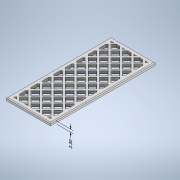
# Autodesk Inventor part: Part_B3
Saved by Autodesk Inventor 2022.6 (Build 266554010, 554A)
## iProperties
Created: 2025-05-15
Part Number: Part_B3
Material: Generic
Document SubType Name: Modeling
Designer: khinm
Density: 1 g/cm^3
Appearance: Default
Author: khinm
Autodesk Inventor part; units mm, degrees
ref_plane "YZ Plane" through (0, 0, 0) normal (1, 0, 0) x (0, 1, 0)
ref_plane "XZ Plane" through (0, 0, 0) normal (0, 1, 0) x (-1, 0, 0)
ref_plane "XY Plane" through (0, 0, 0) normal (0, 0, 1) x (1, 0, 0)
sketch "Sketch1" plane through (0, 0, 0) normal (0, 1, 0) x (-1, 0, 0)
  line L0 (27.4, -64.9) -> (-27.4, -64.9)
  line L1 (-27.4, -64.9) -> (-27.4, 64.9)
  line L2 (-27.4, 64.9) -> (27.4, 64.9)
  line L3 (27.4, 64.9) -> (27.4, -64.9)
  point P0 (0, 0)
  point P1 (27.4, 0)
  point P2 (0, -64.9)
  dimension "d0" = 54.8
  dimension "d1" = 129.8
  constraints: 8 end point, 2 midpoint, 2 parallel, 1 horizontal, 1 horizontal alignment, 1 perpendicular, 1 vertical alignment
  measures "d0" distance of L1.end L2.end
  measures "d1" distance between parallel lines of L2 L0
extrude "Extrusion1" add sketch "Sketch1" along normal mid plane 3.3
sketch "Sketch2" plane through (0, 1.65, 0) normal (0, 1, 0) x (1, 0, 0)
  line L0 (-27.4, -64.9) -> (27.4, -64.9) projected
  line L1 (-27.4, 64.9) -> (-27.4, -64.9) projected
  line L2 (22.4, 59.9) -> (22.4, -59.9)
  line L3 (22.4, -59.9) -> (-22.4, -59.9)
  line L4 (27.4, 64.9) -> (-27.4, 64.9) projected
  line L5 (27.4, -64.9) -> (27.4, 64.9) projected
  line L6 (22.4, 59.9) -> (-22.4, 59.9)
  line L7 (-22.4, -59.9) -> (22.4, -59.9)
  line L8 (22.4, -59.9) -> (22.4, 59.9)
  line L9 (21.2132, -30.0452) -> (22.4, -31.232)
  line L10 (16.2635, -34.9949) -> (21.2132, -39.9447)
  line L11 (-4.9497, -56.2081) -> (-1.2579, -59.9)
  line L12 (-7.0711, -58.3294) -> (-5.5005, -59.9)
  line L13 (14.1421, -37.1162) -> (19.0919, -42.066)
  line L14 (21.2132, -44.1873) -> (22.4, -45.3741)
  line L15 (9.1924, -42.066) -> (14.1421, -47.0157)
  line L16 (16.2635, -49.137) -> (21.2132, -54.0868)
  line L17 (7.0711, -44.1873) -> (12.0208, -49.137)
  line L18 (2.1213, -49.137) -> (7.0711, -54.0868)
  line L19 (9.1924, -56.2081) -> (12.8843, -59.9)
  line L20 (0, -51.2584) -> (4.9497, -56.2081)
  line L21 (7.0711, -58.3294) -> (8.6416, -59.9)
  line L22 (21.2132, -15.903) -> (22.4, -17.0898)
  line L23 (16.2635, -20.8528) -> (21.2132, -25.8025)
  line L24 (14.1421, -22.9741) -> (19.0919, -27.9238)
  line L25 (9.1924, -27.9238) -> (14.1421, -32.8736)
  line L26 (7.0711, -30.0452) -> (12.0208, -34.9949)
  line L27 (2.1213, -34.9949) -> (7.0711, -39.9447)
  line L28 (0, -37.1162) -> (4.9497, -42.066)
  line L29 (-4.9497, -42.066) -> (0, -47.0157)
  line L30 (-7.0711, -44.1873) -> (-2.1213, -49.137)
  line L31 (-12.0208, -49.137) -> (-7.0711, -54.0868)
  line L32 (-21.2132, -44.1873) -> (-16.2635, -49.137)
  line L33 (-14.1421, -51.2584) -> (-9.1924, -56.2081)
  line L34 (-22.4, -52.9) -> (-21.2132, -54.0868)
  line L35 (-19.0919, -56.2081) -> (-15.4, -59.9)
  line L36 (21.2132, -1.7609) -> (22.4, -2.9477)
  line L37 (16.2635, -6.7106) -> (21.2132, -11.6604)
  line L38 (14.1421, -8.832) -> (19.0919, -13.7817)
  line L39 (9.1924, -13.7817) -> (14.1421, -18.7315)
  line L40 (7.0711, -15.903) -> (12.0208, -20.8528)
  line L41 (2.1213, -20.8528) -> (7.0711, -25.8025)
  line L42 (0, -22.9741) -> (4.9497, -27.9238)
  line L43 (-4.9497, -27.9238) -> (0, -32.8736)
  line L44 (-7.0711, -30.0452) -> (-2.1213, -34.9949)
  line L45 (-12.0208, -34.9949) -> (-7.0711, -39.9447)
  line L46 (-21.2132, -30.0452) -> (-16.2635, -34.9949)
  line L47 (-14.1421, -37.1162) -> (-9.1924, -42.066)
  line L48 (-22.4, -38.7579) -> (-21.2132, -39.9447)
  line L49 (-19.0919, -42.066) -> (-14.1421, -47.0157)
  line L50 (22.4, 17.8107) -> (21.2132, 16.6239)
  line L51 (21.2132, 12.3812) -> (22.4, 11.1944)
  line L52 (16.2635, 7.4315) -> (21.2132, 2.4817)
  line L53 (14.1421, 5.3102) -> (19.0919, 0.3604)
  line L54 (9.1924, 0.3604) -> (14.1421, -4.5893)
  line L55 (7.0711, -1.7609) -> (12.0208, -6.7106)
  line L56 (2.1213, -6.7106) -> (7.0711, -11.6604)
  line L57 (0, -8.832) -> (4.9497, -13.7817)
  line L58 (-4.9497, -13.7817) -> (0, -18.7315)
  line L59 (-7.0711, -15.903) -> (-2.1213, -20.8528)
  line L60 (-12.0208, -20.8528) -> (-7.0711, -25.8025)
  line L61 (-21.2132, -15.903) -> (-16.2635, -20.8528)
  line L62 (-14.1421, -22.9741) -> (-9.1924, -27.9238)
  line L63 (-22.4, -24.6157) -> (-21.2132, -25.8025)
  line L64 (-19.0919, -27.9238) -> (-14.1421, -32.8736)
  line L65 (21.2132, 26.5234) -> (22.4, 25.3366)
  line L66 (16.2635, 21.5736) -> (21.2132, 16.6239)
  line L67 (14.1421, 19.4523) -> (19.0919, 14.5026)
  line L68 (9.1924, 14.5026) -> (14.1421, 9.5528)
  line L69 (7.0711, 12.3812) -> (12.0208, 7.4315)
  line L70 (2.1213, 7.4315) -> (7.0711, 2.4817)
  line L71 (0, 5.3102) -> (4.9497, 0.3604)
  line L72 (-4.9497, 0.3604) -> (0, -4.5893)
  line L73 (-7.0711, -1.7609) -> (-2.1213, -6.7106)
  line L74 (-12.0208, -6.7106) -> (-7.0711, -11.6604)
  line L75 (-21.2132, -1.7609) -> (-16.2635, -6.7106)
  line L76 (-14.1421, -8.832) -> (-9.1924, -13.7817)
  line L77 (-22.4, -10.4736) -> (-21.2132, -11.6604)
  line L78 (-19.0919, -13.7817) -> (-14.1421, -18.7315)
  line L79 (-22.4, 59.9) -> (-22.4, -12.8472)
  line L80 (-22.4, -17.0898) -> (-22.4, -59.9)
  line L81 (-22.4, -59.9) -> (-22.4, -17.0898)
  line L82 (-22.4, -12.8472) -> (-22.4, 59.9)
  line L83 (21.2132, 40.6655) -> (22.4, 39.4787)
  line L84 (16.2635, 35.7158) -> (21.2132, 30.766)
  line L85 (14.1421, 33.5944) -> (19.0919, 28.6447)
  line L86 (9.1924, 28.6447) -> (14.1421, 23.6949)
  line L87 (7.0711, 26.5234) -> (12.0208, 21.5736)
  line L88 (2.1213, 21.5736) -> (7.0711, 16.6239)
  line L89 (0, 19.4523) -> (4.9497, 14.5026)
  line L90 (-4.9497, 14.5026) -> (0, 9.5528)
  line L91 (-7.0711, 12.3812) -> (-2.1213, 7.4315)
  line L92 (-12.0208, 7.4315) -> (-7.0711, 2.4817)
  line L93 (-21.2132, 12.3812) -> (-16.2635, 7.4315)
  line L94 (-14.1421, 5.3102) -> (-9.1924, 0.3604)
  line L95 (-22.4, 3.6685) -> (-21.2132, 2.4817)
  line L96 (-19.0919, 0.3604) -> (-14.1421, -4.5893)
  line L97 (16.1209, 59.9) -> (19.0919, 56.929)
  line L98 (21.2132, 54.8076) -> (22.4, 53.6209)
  line L99 (16.2635, 49.8579) -> (21.2132, 44.9082)
  line L100 (14.1421, 47.7366) -> (19.0919, 42.7868)
  line L101 (9.1924, 42.7868) -> (14.1421, 37.8371)
  line L102 (7.0711, 40.6655) -> (12.0208, 35.7158)
  line L103 (2.1213, 35.7158) -> (7.0711, 30.766)
  line L104 (0, 33.5944) -> (4.9497, 28.6447)
  line L105 (-4.9497, 28.6447) -> (0, 23.6949)
  line L106 (-7.0711, 26.5234) -> (-2.1213, 21.5736)
  line L107 (-12.0208, 21.5736) -> (-7.0711, 16.6239)
  line L108 (-21.2132, 26.5234) -> (-16.2635, 21.5736)
  line L109 (-14.1421, 19.4523) -> (-9.1924, 14.5026)
  line L110 (-22.4, 17.8107) -> (-21.2132, 16.6239)
  line L111 (-19.0919, 14.5026) -> (-14.1421, 9.5528)
  line L112 (6.2214, 59.9) -> (7.0711, 59.0503)
  line L113 (9.1924, 56.929) -> (14.1421, 51.9792)
  line L114 (1.9787, 59.9) -> (4.9497, 56.929)
  line L115 (7.0711, 54.8076) -> (12.0208, 49.8579)
  line L116 (2.1213, 49.8579) -> (7.0711, 44.9082)
  line L117 (0, 47.7366) -> (4.9497, 42.7868)
  line L118 (-4.9497, 42.7868) -> (0, 37.8371)
  line L119 (-7.0711, 40.6655) -> (-2.1213, 35.7158)
  line L120 (-12.0208, 35.7158) -> (-7.0711, 30.766)
  line L121 (-21.2132, 40.6655) -> (-16.2635, 35.7158)
  line L122 (-14.1421, 33.5944) -> (-9.1924, 28.6447)
  line L123 (-22.4, 31.9528) -> (-21.2132, 30.766)
  line L124 (-19.0919, 28.6447) -> (-14.1421, 23.6949)
  line L125 (-22.4, 59.9) -> (-6.2214, 59.9)
  line L126 (-1.9787, 59.9) -> (22.4, 59.9)
  line L127 (-7.9208, 59.9) -> (-7.0711, 59.0503)
  line L128 (-4.9497, 56.929) -> (0, 51.9792)
  line L129 (-12.1634, 59.9) -> (-9.1924, 56.929)
  line L130 (-7.0711, 54.8076) -> (-2.1213, 49.8579)
  line L131 (-12.0208, 49.8579) -> (-7.0711, 44.9082)
  line L132 (-21.2132, 54.8076) -> (-16.2635, 49.8579)
  line L133 (-14.1421, 47.7366) -> (-9.1924, 42.7868)
  line L134 (-22.4, 46.0949) -> (-21.2132, 44.9082)
  line L135 (-19.0919, 42.7868) -> (-14.1421, 37.8371)
  line L136 (20.3635, 59.9) -> (21.2132, 59.0503)
  line L137 (22.0629, 59.9) -> (21.2132, 59.0503)
  line L138 (7.9208, 59.9) -> (7.0711, 59.0503)
  line L139 (12.1634, 59.9) -> (9.1924, 56.929)
  line L140 (19.0919, 56.929) -> (14.1421, 51.9792)
  line L141 (21.2132, 54.8076) -> (16.2635, 49.8579)
  line L142 (22.4, 46.0949) -> (21.2132, 44.9082)
  line L143 (-6.2214, 59.9) -> (-7.0711, 59.0503)
  line L144 (-1.9787, 59.9) -> (-4.9497, 56.929)
  line L145 (4.9497, 56.929) -> (0, 51.9792)
  line L146 (7.0711, 54.8076) -> (2.1213, 49.8579)
  line L147 (12.0208, 49.8579) -> (7.0711, 44.9082)
  line L148 (14.1421, 47.7366) -> (9.1924, 42.7868)
  line L149 (19.0919, 42.7868) -> (14.1421, 37.8371)
  line L150 (21.2132, 40.6655) -> (16.2635, 35.7158)
  line L151 (22.4, 31.9528) -> (21.2132, 30.766)
  line L152 (-16.1209, 59.9) -> (-19.0919, 56.929)
  line L153 (-21.2132, 54.8076) -> (-22.4, 53.6209)
  line L154 (-9.1924, 56.929) -> (-14.1421, 51.9792)
  line L155 (-16.2635, 49.8579) -> (-21.2132, 44.9082)
  line L156 (-7.0711, 54.8076) -> (-12.0208, 49.8579)
  line L157 (-2.1213, 49.8579) -> (-7.0711, 44.9082)
  line L158 (0, 47.7366) -> (-4.9497, 42.7868)
  line L159 (4.9497, 42.7868) -> (0, 37.8371)
  line L160 (7.0711, 40.6655) -> (2.1213, 35.7158)
  line L161 (12.0208, 35.7158) -> (7.0711, 30.766)
  line L162 (14.1421, 33.5944) -> (9.1924, 28.6447)
  line L163 (19.0919, 28.6447) -> (14.1421, 23.6949)
  line L164 (21.2132, 26.5234) -> (16.2635, 21.5736)
  line L165 (-14.1421, 47.7366) -> (-19.0919, 42.7868)
  line L166 (-21.2132, 40.6655) -> (-22.4, 39.4787)
  line L167 (-9.1924, 42.7868) -> (-14.1421, 37.8371)
  line L168 (-16.2635, 35.7158) -> (-21.2132, 30.766)
  line L169 (-7.0711, 40.6655) -> (-12.0208, 35.7158)
  line L170 (-2.1213, 35.7158) -> (-7.0711, 30.766)
  line L171 (0, 33.5944) -> (-4.9497, 28.6447)
  line L172 (4.9497, 28.6447) -> (0, 23.6949)
  line L173 (7.0711, 26.5234) -> (2.1213, 21.5736)
  line L174 (12.0208, 21.5736) -> (7.0711, 16.6239)
  line L175 (14.1421, 19.4523) -> (9.1924, 14.5026)
  line L176 (19.0919, 14.5026) -> (14.1421, 9.5528)
  line L177 (21.2132, 12.3812) -> (16.2635, 7.4315)
  line L178 (22.4, 3.6685) -> (21.2132, 2.4817)
  line L179 (-14.1421, 33.5944) -> (-19.0919, 28.6447)
  line L180 (-21.2132, 26.5234) -> (-22.4, 25.3366)
  line L181 (-9.1924, 28.6447) -> (-14.1421, 23.6949)
  line L182 (-16.2635, 21.5736) -> (-21.2132, 16.6239)
  line L183 (-7.0711, 26.5234) -> (-12.0208, 21.5736)
  line L184 (-2.1213, 21.5736) -> (-7.0711, 16.6239)
  line L185 (0, 19.4523) -> (-4.9497, 14.5026)
  line L186 (4.9497, 14.5026) -> (0, 9.5528)
  line L187 (7.0711, 12.3812) -> (2.1213, 7.4315)
  line L188 (12.0208, 7.4315) -> (7.0711, 2.4817)
  line L189 (14.1421, 5.3102) -> (9.1924, 0.3604)
  line L190 (19.0919, 0.3604) -> (14.1421, -4.5893)
  line L191 (21.2132, -1.7609) -> (16.2635, -6.7106)
  line L192 (22.4, -10.4736) -> (21.2132, -11.6604)
  line L193 (-14.1421, 19.4523) -> (-19.0919, 14.5026)
  line L194 (-21.2132, 12.3812) -> (-22.4, 11.1944)
  line L195 (-9.1924, 14.5026) -> (-14.1421, 9.5528)
  line L196 (-16.2635, 7.4315) -> (-21.2132, 2.4817)
  line L197 (-7.0711, 12.3812) -> (-12.0208, 7.4315)
  line L198 (-2.1213, 7.4315) -> (-7.0711, 2.4817)
  line L199 (0, 5.3102) -> (-4.9497, 0.3604)
  line L200 (4.9497, 0.3604) -> (0, -4.5893)
  line L201 (7.0711, -1.7609) -> (2.1213, -6.7106)
  line L202 (12.0208, -6.7106) -> (7.0711, -11.6604)
  line L203 (14.1421, -8.832) -> (9.1924, -13.7817)
  line L204 (19.0919, -13.7817) -> (14.1421, -18.7315)
  line L205 (21.2132, -15.903) -> (16.2635, -20.8528)
  line L206 (22.4, -24.6157) -> (21.2132, -25.8025)
  line L207 (-14.1421, 5.3102) -> (-19.0919, 0.3604)
  line L208 (-21.2132, -1.7609) -> (-22.4, -2.9477)
  line L209 (-9.1924, 0.3604) -> (-14.1421, -4.5893)
  line L210 (-16.2635, -6.7106) -> (-21.2132, -11.6604)
  line L211 (-7.0711, -1.7609) -> (-12.0208, -6.7106)
  line L212 (-2.1213, -6.7106) -> (-7.0711, -11.6604)
  line L213 (0, -8.832) -> (-4.9497, -13.7817)
  line L214 (4.9497, -13.7817) -> (0, -18.7315)
  line L215 (7.0711, -15.903) -> (2.1213, -20.8528)
  line L216 (12.0208, -20.8528) -> (7.0711, -25.8025)
  line L217 (14.1421, -22.9741) -> (9.1924, -27.9238)
  line L218 (-22.4, -12.8472) -> (-22.4, -17.0898)
  line L219 (19.0919, -27.9238) -> (14.1421, -32.8736)
  line L220 (21.2132, -30.0452) -> (16.2635, -34.9949)
  line L221 (22.4, -38.7579) -> (21.2132, -39.9447)
  line L222 (-21.2132, -30.0452) -> (-22.4, -31.232)
  line L223 (-16.2635, -34.9949) -> (-21.2132, -39.9447)
  line L224 (4.9497, -56.2081) -> (1.2579, -59.9)
  line L225 (7.0711, -58.3294) -> (5.5005, -59.9)
  line L226 (-14.1421, -8.832) -> (-19.0919, -13.7817)
  line L227 (-21.2132, -15.903) -> (-22.4, -17.0898)
  line L228 (-9.1924, -13.7817) -> (-14.1421, -18.7315)
  line L229 (-16.2635, -20.8528) -> (-21.2132, -25.8025)
  line L230 (-7.0711, -15.903) -> (-12.0208, -20.8528)
  line L231 (-14.1421, -22.9741) -> (-19.0919, -27.9238)
  line L232 (-2.1213, -20.8528) -> (-7.0711, -25.8025)
  line L233 (-9.1924, -27.9238) -> (-14.1421, -32.8736)
  line L234 (0, -22.9741) -> (-4.9497, -27.9238)
  line L235 (-7.0711, -30.0452) -> (-12.0208, -34.9949)
  line L236 (4.9497, -27.9238) -> (0, -32.8736)
  line L237 (-2.1213, -34.9949) -> (-7.0711, -39.9447)
  line L238 (7.0711, -30.0452) -> (2.1213, -34.9949)
  line L239 (0, -37.1162) -> (-4.9497, -42.066)
  line L240 (12.0208, -34.9949) -> (7.0711, -39.9447)
  line L241 (4.9497, -42.066) -> (0, -47.0157)
  line L242 (14.1421, -37.1162) -> (9.1924, -42.066)
  line L243 (7.0711, -44.1873) -> (2.1213, -49.137)
  line L244 (19.0919, -42.066) -> (14.1421, -47.0157)
  line L245 (12.0208, -49.137) -> (7.0711, -54.0868)
  line L246 (21.2132, -44.1873) -> (16.2635, -49.137)
  line L247 (14.1421, -51.2584) -> (9.1924, -56.2081)
  line L248 (22.4, -52.9) -> (21.2132, -54.0868)
  line L249 (19.0919, -56.2081) -> (15.4, -59.9)
  line L250 (-14.1421, -37.1162) -> (-19.0919, -42.066)
  line L251 (-21.2132, -44.1873) -> (-22.4, -45.3741)
  line L252 (-9.1924, -42.066) -> (-14.1421, -47.0157)
  line L253 (-16.2635, -49.137) -> (-21.2132, -54.0868)
  line L254 (-7.0711, -44.1873) -> (-12.0208, -49.137)
  line L255 (-2.1213, -49.137) -> (-7.0711, -54.0868)
  line L256 (-9.1924, -56.2081) -> (-12.8843, -59.9)
  line L257 (0, -51.2584) -> (-4.9497, -56.2081)
  line L258 (-7.0711, -58.3294) -> (-8.6416, -59.9)
  line L259 (-21.2132, -58.3294) -> (-19.6426, -59.9)
  line L260 (-14.1421, -51.2584) -> (-19.0919, -56.2081)
  line L261 (-21.2132, -58.3294) -> (-22.4, -59.5162)
  line L262 (21.2132, -58.3294) -> (19.6426, -59.9)
  line L263 (14.1421, -51.2584) -> (19.0919, -56.2081)
  line L264 (21.2132, -58.3294) -> (22.4, -59.5162)
  line L265 (-20.3635, 59.9) -> (-21.2132, 59.0503)
  line L266 (-22.0629, 59.9) -> (-21.2132, 59.0503)
  line L267 (-19.0919, 56.929) -> (-14.1421, 51.9792)
  point P0 (-27.4, 0)
  point P1 (-22.4, 0)
  point P2 (0, 64.9)
  point P3 (22.4, 0)
  dimension "d51" = 5
  dimension "d52" = 5
  dimension "d53" = 7
  dimension "d54" = 7
  dimension "d78" = 3
  dimension "d79" = 3
  dimension "d80" = 3
  dimension "d81" = 3
  constraints: 765 parallel, 522 end point, 35 point on line, 4 horizontal, 3 vertical, 2 midpoint, 1 horizontal alignment, 34 other
  measures "d51" distance between parallel lines of L0 L3
  measures "d53" distance of L35.end L3.end
  measures "d54" distance of L34.start L3.end
  measures "d78" distance between parallel lines of L97 L136
  measures "d79" distance between parallel lines of L35 L259
  measures "d80" distance between parallel lines of L249 L262
  measures "d81" distance between parallel lines of L152 L265
extrude "Extrusion2" cut sketch "Sketch2" against normal up to surface (3.3 mm away) contours L2 L142 L99 L141 L98 | L137 L136 L6 | L2 L151 L84 L150 L83 | L97 L140 L113 L139 L6 | L2 L50 L66 L164 L65 | L138 L112 L6 | L2 L178 L52 L177 L51 | L114 L145 L128 L144 L6 | L2 L192 L37 L191 L36 | L143 L127 L6 | L2 L206 L23 L205 L22 | L129 L154 L267 L152 L6 | L2 L221 L10 L220 L9 | L265 L266 L6 | L2 L248 L16 L246 L14 | L153 L132 L155 L134 L79 | L2 L3 L262 L264 | L166 L121 L168 L123 L79 | L3 L19 L247 L263 L249 | L180 L108 L182 L110 L79 | L3 L225 L21 | L194 L93 L196 L95 L79 | L3 L11 L257 L20 L224 | L208 L75 L210 L77 L79 | L3 L258 L12 | L227 L61 L229 L63 L80 | L3 L35 L260 L33 L256 | L222 L46 L223 L48 L80 | L3 L80 L261 L259 | L251 L32 L253 L34 L80 | L13 L244 L15 L242 | L17 L245 L18 L243 | L24 L219 L25 L217 | L26 L240 L27 L238 | L28 L241 L29 L239 | L30 L255 L31 L254 | L38 L204 L39 L203 | L40 L216 L41 L215 | L42 L236 L43 L234 | L44 L237 L45 L235 | L47 L252 L49 L250 | L53 L190 L54 L189 | L55 L202 L56 L201 | L57 L214 L58 L213 | L59 L232 L60 L230 | L62 L233 L64 L231 | L67 L176 L68 L175 | L69 L188 L70 L187 | L71 L200 L72 L199 | L73 L212 L74 L211 | L76 L228 L78 L226 | L85 L163 L86 L162 | L87 L174 L88 L173 | L89 L186 L90 L185 | L91 L198 L92 L197 | L94 L209 L96 L207 | L100 L149 L101 L148 | L102 L161 L103 L160 | L104 L172 L105 L171 | L106 L184 L107 L183 | L109 L195 L111 L193 | L115 L147 L116 L146 | L117 L159 L118 L158 | L119 L170 L120 L169 | L122 L181 L124 L179 | L130 L157 L131 L156 | L133 L167 L135 L165
fillet "Fillet1" radius 1 4 edges at (27.4, 1.65, 0) (0, 1.65, 64.9) (-27.4, 1.65, 0) (0, 1.65, -64.9)
chamfer "Chamfer2" distance 0.4 angle 45 73 edges at (-20.7883, 1.65, -59.4751) (-21.6381, 1.65, -59.4751) (-21.2132, 1.65, -59.9) (-17.6064, 1.65, -58.4145) (-11.6673, 1.65, -54.4541) (-10.6779, 1.65, -58.4145) (-16.617, 1.65, -54.4541) (-14.1421, 1.65, -59.9) (-7.0711, 1.65, -59.9) (-6.6462, 1.65, -59.4751) (-7.4959, 1.65, -59.4751) (-2.4749, 1.65, -54.4541) (4.5962, 1.65, -47.383) (11.6673, 1.65, -40.312) (18.7383, 1.65, -33.2409) (16.617, 1.65, -45.2617) (9.5459, -1.65, -52.3328) (9.5459, 1.65, -52.3328) (3.4642, 1.65, -58.4145) (6.6462, 1.65, -59.4751) (11.6673, 1.65, -54.4541) (18.7383, 1.65, -47.383) (21.8066, 1.65, -54.2142) (17.6064, 1.65, -58.4145) (20.7883, 1.65, -59.4751) (-4.5962, 1.65, -52.3328) (2.4749, 1.65, -45.2617) (9.5459, 1.65, -38.1906) (16.617, 1.65, -31.1196) (21.8066, 1.65, -25.93) (-9.5459, 1.65, -47.383) (-2.4749, 1.65, -40.312) (4.5962, 1.65, -33.2409) (11.6673, 1.65, -26.1698) (18.7383, 1.65, -19.0988) (-18.7383, 1.65, -52.3328) (-11.6673, 1.65, -45.2617) (-4.5962, 1.65, -38.1906) (2.4749, 1.65, -31.1196) (9.5459, 1.65, -24.0485) (-3.4642, 1.65, -58.4145) (-9.5459, 1.65, -52.3328) (-16.617, 1.65, -45.2617) (-18.7383, 1.65, -47.383) (-21.8066, 1.65, -45.5016) (-21.8066, 1.65, -54.2142) (-4.5962, 1.65, -47.383) (2.4749, 1.65, -54.4541) (7.4959, 1.65, -59.4751) (10.6779, 1.65, -58.4145) (4.5962, 1.65, -52.3328) (-2.4749, 1.65, -45.2617) (2.4749, 1.65, -40.312) (9.5459, 1.65, -47.383) (16.617, 1.65, -54.4541) (21.6381, 1.65, -59.4751) (18.7383, 1.65, -52.3328) (11.6673, 1.65, -45.2617) (4.5962, 1.65, -38.1906) (9.5459, 1.65, -33.2409) (16.617, 1.65, -40.312) (21.8066, 1.65, -45.5016) (18.7383, 1.65, -38.1906) (11.6673, 1.65, -31.1196) (21.8066, 1.65, -40.0721) (0, 1.65, -59.9) (7.0711, 1.65, -59.9) (14.1421, 1.65, -59.9) (21.2132, 1.65, -59.9) (22.4, 1.65, -49.8579) (22.4, 1.65, -35.7158) (21.8066, 1.65, -31.3594) (-21.8066, 1.65, -40.0721)
chamfer "Chamfer3" distance 0.4 angle 45 53 edges at (-21.3546, 1.65, -40.8069) (-18.7383, 1.65, -38.1906) (-19.2333, 1.65, -42.9283) (-16.617, 1.65, -40.312) (-9.5459, 1.65, -33.2409) (-2.4749, 1.65, -26.1698) (4.5962, 1.65, -19.0988) (11.6673, 1.65, -12.0277) (16.617, 1.65, -16.9774) (21.8066, 1.65, -11.7878) (-18.7383, 1.65, -33.2409) (-9.051, 1.65, -42.9283) (-11.6673, 1.65, -40.312) (-21.8066, 1.65, -31.3594) (-16.617, 1.65, -31.1196) (-6.9296, 1.65, -40.8069) (-9.5459, 1.65, -38.1906) (-21.8066, 1.65, -25.93) (-18.7383, 1.65, -19.0988) (-11.6673, 1.65, -26.1698) (-1.9799, 1.65, -35.8572) (-4.5962, 1.65, -33.2409) (0.1414, 1.65, -33.7359) (-2.4749, 1.65, -31.1196) (-9.5459, 1.65, -24.0485) (-16.617, 1.65, -16.9774) (-4.5962, 1.65, -19.0988) (5.0912, 1.65, -28.7861) (2.4749, 1.65, -26.1698) (7.2125, 1.65, -26.6648) (4.5962, 1.65, -24.0485) (-2.4749, 1.65, -16.9774) (-11.6673, 1.65, -12.0277) (-9.5459, 1.65, -9.9064) (2.4749, 1.65, -12.0277) (12.1622, 1.65, -21.7151) (9.5459, 1.65, -19.0988) (14.0007, 1.65, -23.5535) (16.617, 1.65, -26.1698) (19.2333, 1.65, -28.7861) (21.3546, 1.65, -26.6648) (18.7383, 1.65, -24.0485) (16.122, 1.65, -21.4322) (11.6673, 1.65, -16.9774) (4.5962, 1.65, -9.9064) (-16.617, 1.65, -26.1698) (-9.5459, 1.65, -19.0988) (-2.4749, 1.65, -12.0277) (4.5962, 1.65, -4.9566) (-11.6673, 1.65, -31.1196) (-4.5962, 1.65, -24.0485) (2.4749, 1.65, -16.9774) (9.5459, 1.65, -9.9064)
chamfer "Chamfer4" distance 0.4 angle 45 75 edges at (-4.5962, 1.65, -4.9566) (-11.6673, 1.65, 2.1144) (-18.7383, 1.65, 9.1855) (-18.7383, 1.65, -9.9064) (-19.2333, 1.65, -14.644) (-16.617, 1.65, -12.0277) (-14.0007, 1.65, -9.4114) (-12.1622, 1.65, -7.5729) (-9.5459, 1.65, -4.9566) (-2.4749, 1.65, 2.1144) (4.5962, 1.65, 9.1855) (11.6673, 1.65, 16.2566) (18.7383, 1.65, 23.3277) (21.8066, 1.65, 16.4964) (16.617, 1.65, 11.3068) (9.5459, 1.65, 4.2358) (2.4749, 1.65, -2.8353) (-7.2125, 1.65, -12.5227) (-4.5962, 1.65, -9.9064) (-14.2836, 1.65, -19.5937) (-11.6673, 1.65, -16.9774) (-9.051, 1.65, -14.3611) (-21.0718, 1.65, -16.4825) (-21.8066, 1.65, -17.2173) (14.0007, 1.65, -9.4114) (16.617, 1.65, -12.0277) (19.2333, 1.65, -14.644) (21.0718, 1.65, -16.4825) (21.8066, 1.65, -17.2173) (21.3546, 1.65, -12.5227) (18.7383, 1.65, -9.9064) (6.9296, 1.65, -2.3403) (9.5459, 1.65, -4.9566) (12.1622, 1.65, -7.5729) (11.6673, 1.65, -2.8353) (16.617, 1.65, -2.8353) (16.617, 1.65, 2.1144) (11.6673, 1.65, 2.1144) (18.7383, 1.65, 4.2358) (21.8066, 1.65, 2.3543) (18.7383, 1.65, 9.1855) (21.8066, 1.65, 11.067) (22.4, 1.65, 6.7106) (18.7383, 1.65, -4.9566) (21.8066, 1.65, -3.0751) (22.4, 1.65, -11.4773) (22.4, 1.65, -7.4315) (2.4749, 1.65, 2.1144) (4.5962, 1.65, 4.2358) (9.5459, 1.65, 9.1855) (11.6673, 1.65, 11.3068) (16.617, 1.65, 16.2566) (18.7383, 1.65, 18.3779) (-21.8066, 1.65, -11.7878) (-21.8066, 1.65, -3.0751) (-18.7383, 1.65, -4.9566) (-16.617, 1.65, -2.8353) (-21.8066, 1.65, 2.3543) (-18.7383, 1.65, 4.2358) (-21.8066, 1.65, 11.067) (-16.617, 1.65, 11.3068) (-16.617, -1.65, 11.3068) (-9.5459, 1.65, 4.2358) (-9.5459, 1.65, 9.1855) (-11.6673, 1.65, 11.3068) (-4.5962, 1.65, 9.1855) (-4.5962, 1.65, 4.2358) (-2.4749, 1.65, 11.3068) (2.4749, 1.65, 16.2566) (2.4749, 1.65, 11.3068) (-2.4749, 1.65, 16.2566) (4.5962, 1.65, 18.3779) (9.5459, 1.65, 18.3779) (-16.617, 1.65, 2.1144) (-11.6673, 1.65, -2.8353)
chamfer "Chamfer5" distance 0.4 angle 45 49 edges at (-9.051, 1.65, 13.6403) (-11.6673, 1.65, 16.2566) (-19.2333, 1.65, 13.6403) (-16.617, 1.65, 16.2566) (-18.7383, 1.65, 18.3779) (-21.8066, 1.65, 16.4964) (-11.6673, 1.65, 25.449) (-9.5459, 1.65, 23.3277) (-9.5459, 1.65, 18.3779) (-4.5962, 1.65, 18.3779) (-4.5962, 1.65, 23.3277) (-2.4749, 1.65, 25.449) (2.4749, 1.65, 25.449) (-2.4749, 1.65, 30.3987) (2.4749, 1.65, 30.3987) (4.5962, 1.65, 32.52) (9.5459, 1.65, 32.52) (9.5459, 1.65, 37.4698) (4.5962, 1.65, 37.4698) (11.6673, 1.65, 30.3987) (11.6673, 1.65, 25.449) (12.1622, 1.65, 20.7114) (9.5459, 1.65, 23.3277) (1.9799, 1.65, 20.7114) (4.5962, 1.65, 23.3277) (16.617, 1.65, 25.449) (16.617, 1.65, 30.3987) (18.7383, 1.65, 32.52) (21.8066, 1.65, 30.6386) (18.7383, 1.65, 37.4698) (21.8066, 1.65, 39.3513) (16.617, 1.65, 39.5911) (11.6673, 1.65, 44.5409) (11.6673, 1.65, 39.5911) (16.617, 1.65, 44.5409) (18.7383, 1.65, 46.6622) (21.8066, 1.65, 44.7807) (-18.7383, 1.65, 23.3277) (-16.617, 1.65, 25.449) (-11.6673, 1.65, 30.3987) (-9.5459, 1.65, 32.52) (-4.5962, 1.65, 37.4698) (-2.4749, 1.65, 39.5911) (2.4749, 1.65, 44.5409) (4.5962, 1.65, 46.6622) (-21.8066, 1.65, 30.6386) (-18.7383, 1.65, 37.4698) (-11.6673, 1.65, 44.5409) (-16.617, 1.65, 39.5911)
chamfer "Chamfer6" distance 0.4 angle 45 58 edges at (-19.2333, 1.65, 27.7825) (-16.617, 1.65, 30.3987) (-14.0007, 1.65, 33.015) (-21.3546, 1.65, 29.9038) (-18.7383, 1.65, 32.52) (-16.1221, 1.65, 35.1363) (-21.8066, 1.65, 25.2091) (-21.0718, 1.65, 25.9439) (-12.1622, 1.65, 34.8535) (-9.5459, 1.65, 37.4698) (-6.9297, 1.65, 40.086) (-9.051, 1.65, 42.2074) (-11.6673, 1.65, 39.5911) (-14.2835, 1.65, 36.9748) (-5.0911, 1.65, 41.9246) (-2.4749, 1.65, 44.5409) (0.1414, 1.65, 47.1571) (-4.5962, 1.65, 46.6622) (1.9799, 1.65, 48.9957) (4.5962, 1.65, 51.6119) (2.4749, 1.65, 53.7332) (9.5459, 1.65, 51.6119) (11.6673, 1.65, 53.7332) (16.617, 1.65, 53.7332) (16.1221, 1.65, 48.9957) (18.7383, 1.65, 51.6119) (6.9297, 1.65, 44.0459) (9.5459, 1.65, 46.6622) (2.4749, -1.65, 39.5911) (-0.1414, 1.65, 36.9748) (2.4749, 1.65, 39.5911) (5.0911, 1.65, 42.2074) (-7.2125, 1.65, 29.9038) (-4.5962, 1.65, 32.52) (-1.9799, 1.65, 35.1363) (-14.0007, 1.65, 47.1571) (-16.617, 1.65, 44.5409) (-19.2333, 1.65, 41.9246) (-21.0718, 1.65, 40.086) (-21.8066, 1.65, 39.3513) (-9.5459, 1.65, 51.6119) (-3.1038, 1.65, 58.0541) (-4.5962, 1.65, 51.6119) (-2.4749, 1.65, 53.7332) (-9.5459, 1.65, 46.6622) (3.1038, 1.65, 58.0541) (21.8066, 1.65, 53.4934) (11.0383, 1.65, 58.0541) (17.2459, 1.65, 58.0541) (-18.7383, -1.65, 51.6119) (-18.7383, 1.65, 51.6119) (-18.7383, 1.65, 46.6622) (-21.8066, 1.65, 44.7807) (-21.8066, 1.65, 53.4934) (-16.617, 1.65, 53.7332) (-17.2459, 1.65, 58.0541) (-11.6673, 1.65, 53.7332) (-11.0383, 1.65, 58.0541)
chamfer "Chamfer7" distance 0.4 angle 45 23 edges at (-21.8066, 1.65, 58.9228) (-7.8563, 1.65, 59.1147) (-6.2858, 1.65, 59.1147) (6.2858, 1.65, 59.1147) (7.8563, 1.65, 59.1147) (20.4279, 1.65, 59.1147) (21.8066, 1.65, 58.9228) (21.0213, 1.65, 59.9) (22.4, 1.65, 59.7081) (-21.0213, 1.65, 59.9) (-20.4279, 1.65, 59.1147) (-22.4, 1.65, 59.7081) (-15.6825, 1.65, 59.9) (-14.1421, 1.65, 59.9) (-12.6018, 1.65, 59.9) (-7.0711, 1.65, 59.9) (-1.5404, 1.65, 59.9) (0, 1.65, 59.9) (1.5404, 1.65, 59.9) (7.0711, 1.65, 59.9) (12.6018, 1.65, 59.9) (14.1421, 1.65, 59.9) (15.6825, 1.65, 59.9)
chamfer "Chamfer8" distance 0.4 angle 45 23 edges at (22.4, 1.65, 45.0913) (22.4, 1.65, 49.137) (22.4, 1.65, 53.1825) (22.4, 1.65, 30.9492) (22.4, 1.65, 34.9949) (22.4, 1.65, 39.0406) (22.4, 1.65, 20.8528) (22.4, 1.65, 16.807) (-22.4, 1.65, 45.0916) (-22.4, 1.65, 49.137) (-22.4, 1.65, 53.1825) (-22.4, 1.65, 39.0404) (-22.4, 1.65, 34.9949) (-22.4, 1.65, 30.9492) (-22.4, 1.65, 24.8982) (-22.4, 1.65, 20.8528) (-22.4, 1.65, 16.8071) (-22.4, 1.65, 2.6648) (-22.4, 1.65, 6.7106) (-22.4, 1.65, 10.7564) (-22.4, 1.65, -11.4773) (-22.4, 1.65, -7.4315) (-22.4, 1.65, -3.3857)
chamfer "Chamfer9" distance 0.4 angle 45 12 edges at (-22.4, 1.65, -17.5278) (-22.4, 1.65, -21.5736) (-22.4, 1.65, -25.6194) (-22.4, 1.65, -39.7616) (-22.4, 1.65, -35.7158) (-22.4, 1.65, -31.67) (-22.4, 1.65, -45.8121) (-22.4, 1.65, -49.8579) (-22.4, 1.65, -53.9037) (22.4, 1.65, -17.5278) (22.4, 1.65, -21.5736) (22.4, 1.65, -25.6194)
body "Solid1"
